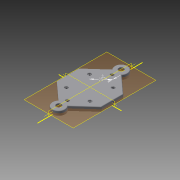
# Autodesk Inventor part: ChassisOberTeil
Saved by Autodesk Inventor 2015 (Build 190159000, 159)
## iProperties
Created: 2018-11-02
Part Number: ChassisOberTeil
Material: Generisch
Document SubType Name: Modeling
Designer: Boris
Density: 1 g/cm^3
Appearance: Vorgabe
Author: Boris
Autodesk Inventor part; units mm, degrees
sketch "Skizze1" plane through (0, 0, 0) normal (0, 0, 1) x (1, 0, 0)
  line L0 (-35, 17.188) -> (-35, -17.188)
  line L1 (35, 17.188) -> (35, -17.188)
  line L2 (-35, 17.188) -> (-7.4001, 42.274)
  line L3 (35, 17.188) -> (7.4001, 42.274)
  line L4 (-35, -17.188) -> (-7.4001, -42.274)
  line L5 (7.4001, -42.274) -> (35, -17.188)
  arc A0 (-7.4001, -42.274) -> (7.4001, -42.274) centre (0, -49) ccw
  arc A1 (7.4001, 42.274) -> (-7.4001, 42.274) centre (0, 49) ccw
  point P0 (0, 0)
  dimension "d2" = 34.376
  dimension "d3" = 20
  dimension "d4" = 20
  constraints: 12 end point, 4 point on circle, 2 centre point, 1 parallel, 1 vertical
  measures "d2" distance of L0.start L0.end
  measures "d3" diameter of A0
  measures "d4" diameter of A1
extrude "Extrusion1" add sketch "Skizze1" along normal mid plane 7
sketch "Skizze2" plane through (0, 0, -3.5) normal (0, 0, -1) x (-1, 0, 0)
  arc A0 (-7.4001, -42.274) -> (7.4001, -42.274) centre (0, -49) ccw projected
  arc A1 (7.4001, 42.274) -> (-7.4001, 42.274) centre (0, 49) ccw projected
  circle A2 centre (0, 49) radius 7
  circle A3 centre (0, -49) radius 7
  point P0 (0, 0)
  dimension "d7" = 14
  dimension "d8" = 14
  constraints: 2 centre point, 2 coincident
  measures "d7" diameter of A2
  measures "d8" diameter of A3
extrude "Extrusion2" cut sketch "Skizze2" against normal blind 5
sketch "Skizze3" plane through (0, 0, -3.5) normal (0, 0, -1) x (-1, 0, 0)
  circle A0 centre (0, 49) radius 7 projected
  circle A1 centre (0, 35) radius 1.5
  line L0 (35, 17.188) -> (7.4001, 42.274) projected
  circle A2 centre (18.5001, 18.185) radius 1.5
  line L1 (49, 0) -> (-49, 0) projected
  circle A3 centre (0, -35) radius 1.5
  circle A4 centre (18.5001, -18.185) radius 1.5
  line L2 (0, -82.6) -> (0, 82.6) projected
  circle A5 centre (-18.5001, 18.185) radius 1.5
  circle A6 centre (-18.5001, -18.185) radius 1.5
  point P0 (0, 0)
  dimension "d11" = 3
  dimension "d14" = 25
  constraints: 6 centre point, 4 symmetric about line, 7 other
  measures "d11" diameter of A1
  measures "d14" distance of A1.centre A2.centre
extrude "Extrusion3" cut sketch "Skizze3" against normal blind 7 contours A3 L2 | L2 A3 | A1 L2 | L2 A1 | A2 | A4
thread "Gewinde1" size "M3x0.5" class "6H" standard "ANSI Metric M Profile" full length
thread "Gewinde2" size "M3x0.5" class "6H" standard "ANSI Metric M Profile" full length
thread "Gewinde3" size "M3x0.5" class "6H" standard "ANSI Metric M Profile" full length
thread "Gewinde4" size "M3x0.5" class "6H" standard "ANSI Metric M Profile" full length
sketch "Skizze4" plane through (0, 0, 3.5) normal (0, 0, 1) x (1, 0, 0)
  circle A0 centre (0, 49) radius 7 projected
  circle A1 centre (0, -49) radius 7 projected
  circle A2 centre (0, 49) radius 4
  circle A3 centre (0, -49) radius 4
  point P0 (0, 0)
  dimension "d29" = 8
  dimension "d30" = 8
  constraints: 2 centre point, 2 coincident
  measures "d29" diameter of A2
  measures "d30" diameter of A3
extrude "Extrusion4" cut sketch "Skizze4" against normal blind 2 contours A2 | A3
fillet "Rundung1" radius 1 1 edges at (7, 49, 1.5)
fillet "Rundung2" radius 1 1 edges at (7, -49, 1.5)
fillet "Rundung4" radius 1 4 edges at (35, 17.188, 0) (35, -17.188, 0) (-35, -17.188, 0) (-35, 17.188, 0)
extrude "Extrusion5" cut sketch "Skizze3" against normal blind 7 contours A5 | A6
thread "Gewinde5" size "M3x0.5" class "6H" standard "ANSI Metric M Profile" full length
thread "Gewinde6" size "M3x0.5" class "6H" standard "ANSI Metric M Profile" full length
sketch "Skizze5" plane through (0, 0, 3.5) normal (0, 0, 1) x (1, 0, 0)
  circle A0 centre (-18.5001, -18.185) radius 1.5 projected
  circle A1 centre (0, -35) radius 1.5 projected
  circle A2 centre (18.5001, -18.185) radius 1.5 projected
  circle A3 centre (18.5001, 18.185) radius 1.5 projected
  circle A4 centre (0, 35) radius 1.5 projected
  circle A5 centre (-18.5001, 18.185) radius 1.5 projected
  line L0 (-21.0001, 18) -> (-19.9103, 20.2575)
  line L1 (-19.9103, 20.2575) -> (-17.4103, 20.4425)
  line L2 (-17.4103, 20.4425) -> (-16.0001, 18.3699)
  line L3 (-16.0001, 18.3699) -> (-17.0899, 16.1124)
  line L4 (-17.0899, 16.1124) -> (-19.5899, 15.9274)
  line L5 (-19.5899, 15.9274) -> (-21.0001, 18)
  line L6 (-49, 0) -> (49, 0) projected
  line L7 (0, 82.6) -> (0, -82.6) projected
  line L8 (21.0001, 18) -> (19.9103, 20.2575)
  line L9 (19.9103, 20.2575) -> (17.4103, 20.4425)
  line L10 (17.4103, 20.4425) -> (16.0001, 18.3699)
  line L11 (16.0001, 18.3699) -> (17.0899, 16.1124)
  line L12 (17.0899, 16.1124) -> (19.5899, 15.9274)
  line L13 (19.5899, 15.9274) -> (21.0001, 18)
  line L14 (-21.0001, -18) -> (-19.9103, -20.2575)
  line L15 (-19.9103, -20.2575) -> (-17.4103, -20.4425)
  line L16 (-17.4103, -20.4425) -> (-16.0001, -18.3699)
  line L17 (-16.0001, -18.3699) -> (-17.0899, -16.1124)
  line L18 (-17.0899, -16.1124) -> (-19.5899, -15.9274)
  line L19 (-19.5899, -15.9274) -> (-21.0001, -18)
  line L20 (21.0001, -18) -> (19.9103, -20.2575)
  line L21 (19.5899, -15.9274) -> (21.0001, -18)
  line L22 (17.0899, -16.1124) -> (19.5899, -15.9274)
  line L23 (16.0001, -18.3699) -> (17.0899, -16.1124)
  line L24 (17.4103, -20.4425) -> (16.0001, -18.3699)
  line L25 (19.9103, -20.2575) -> (17.4103, -20.4425)
  line L26 (-2.5, -35) -> (-1.25, -32.8349)
  line L27 (-1.25, -32.8349) -> (1.25, -32.8349)
  line L28 (1.25, -32.8349) -> (2.5, -35)
  line L29 (2.5, -35) -> (1.25, -37.1651)
  line L30 (1.25, -37.1651) -> (-1.25, -37.1651)
  line L31 (-1.25, -37.1651) -> (-2.5, -35)
  line L32 (-2.5, 35) -> (-1.25, 32.8349)
  line L33 (-1.25, 32.8349) -> (1.25, 32.8349)
  line L34 (1.25, 32.8349) -> (2.5, 35)
  line L35 (2.5, 35) -> (1.25, 37.1651)
  line L36 (1.25, 37.1651) -> (-1.25, 37.1651)
  line L37 (-1.25, 37.1651) -> (-2.5, 35)
  point P0 (0, 0)
  constraints: 72 end point, 24 symmetric about line, 26 other
extrude "Extrusion6" cut sketch "Skizze5" against normal blind 2 contours A1 L7 L27 L28 L29 L30 | A1 L7 L30 L31 L26 L27 | L33 L32 L37 L36 L7 A4 | L7 A4 L36 L35 L34 L33 | L0 L1 L2 L3 L4 L5 | L13 L12 L11 L10 L9 L8 | L19 L18 L17 L16 L15 L14 | L20 L25 L24 L23 L22 L21
fillet "Rundung5" radius 1 12 edges at (0, 59, 3.5) (0, -59, 3.5) (-34.9145, -17.1502, 3.5) (-35, 0, 3.5) (-34.9145, 17.1502, 3.5) (-21.0363, 29.8798, 3.5) (-21.0363, -29.8798, 3.5) (34.9145, -17.1502, 3.5) (35, 0, 3.5) (34.9145, 17.1502, 3.5) (21.0363, 29.8798, 3.5) (21.0363, -29.8798, 3.5)
fillet "Rundung6" radius 1 35 edges at (1.875, 36.0825, 3.5) (0, 37.1651, 3.5) (-1.875, 33.9175, 3.5) (-1.875, 36.0825, 3.5) (0, 32.8349, 3.5) (1.875, 33.9175, 3.5) (16.7052, 19.4062, 3.5) (18.6603, 20.35, 3.5) (20.4552, 19.1288, 3.5) (20.295, 16.9637, 3.5) (18.3399, 16.0199, 3.5) (16.545, 17.2412, 3.5) (-16.545, 17.2412, 3.5) (-18.3399, 16.0199, 3.5) (-20.295, 16.9637, 3.5) (-20.4552, 19.1288, 3.5) (-18.6603, 20.35, 3.5) (-16.7052, 19.4062, 3.5) (-20.4552, -19.1288, 3.5) (-18.6603, -20.35, 3.5) (-16.7052, -19.4062, 3.5) (-16.545, -17.2412, 3.5) (-18.3399, -16.0199, 3.5) (-20.295, -16.9637, 3.5) (-1.875, -33.9175, 3.5) (-1.875, -36.0825, 3.5) (0, -37.1651, 3.5) (1.875, -36.0825, 3.5) (1.875, -33.9175, 3.5) (0, -32.8349, 3.5) (16.7052, -19.4062, 3.5) (16.545, -17.2412, 3.5) (18.3399, -16.0199, 3.5) (20.295, -16.9637, 3.5) (18.6603, -20.35, 3.5)
fillet "Rundung6" radius 1 1 edges at (20.4552, -19.1288, 3.5)
